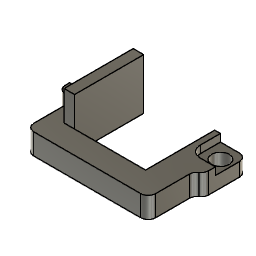
GB DMG - Jack Spacer v15 (Autodesk Fusion 360 design; units mm, degrees)
Autodesk Fusion 360 part; units mm, degrees
sketch "Boceto1" plane through (0, 0, 0) normal (0, 0, 1) x (1, 0, 0)
  line L0 (0, 0) -> (-8.15, 0)
  line L1 (-8.15, 0) -> (-8.15, 6.5)
  line L2 (-8.15, 6.5) -> (-10.45, 6.5)
  line L3 (-10.45, 6.5) -> (-10.45, 12.3)
  line L4 (-10.45, 12.3) -> (-4.75, 12.3)
  line L5 (0, 3.05) -> (-4.75, 3.05)
  line L6 (-4.75, 3.05) -> (-4.75, 12.3)
  line L7 (0, 3.05) -> (0, 0)
  line L8 (4.75, 3.05) -> (4.75, 12.3)
  line L9 (8.15, 6.5) -> (10.45, 6.5)
  line L10 (8.15, 0) -> (8.15, 6.5)
  line L11 (10.45, 12.3) -> (4.75, 12.3)
  line L12 (0, 3.05) -> (4.75, 3.05)
  line L13 (10.45, 6.5) -> (10.45, 12.3)
  line L14 (0, 3.05) -> (0, 0)
  line L15 (0, 0) -> (8.15, 0)
  dimension "d2" = 5.8
  dimension "d3" = 2.3
  dimension "d5" = 8.15
  dimension "d7" = 3.4
  dimension "d8" = 3.05
  dimension "d22" = 9.25
  constraint coincident L0.start L7.end
  constraint horizontal L0
  constraint perpendicular L0 L1
  constraint perpendicular L1 L2
  constraint perpendicular L0 L3
  constraint perpendicular L1 L4
  constraint parallel L4 L5
  constraint perpendicular L4 L6
  constraint perpendicular L0 L7
  constraint symmetric L0.start L7 L14.end
  constraint symmetric L0.end L7 L10.start
  constraint symmetric L1.end L7 L9.start
  constraint symmetric L2.end L7 L9.end
  constraint symmetric L3.end L7 L11.start
  constraint symmetric L5.start L7 L12.start
  constraint symmetric L5.end L7 L8.start
  constraint symmetric L4.end L7 L8.end
  measures "d2" distance of L2.end L3.end
  measures "d3" distance of L1.end L2.end
  measures "d5" distance of L0.start L0.end
  measures "d7" horizontal distance of L1.end L4.end
  measures "d8" distance of L0.start L5.start
  measures "d22" distance of L5.end L4.end
extrude "Extruir1" add sketch "Boceto1" along normal blind 2.8
extrude "Extruir7" cut 1 faces at (10.45, 8.4333, 0.9333) along direction (-1, 0, 0) blind 0.5
sketch "Boceto2" plane through (0, 0, 2.8) normal (0, 0, 1) x (-1, 0, 0)
  line L0 (8.15, 0) -> (-8.15, 0)
  line L1 (-8.15, 0) -> (-8.15, -6.5)
  line L2 (-8.15, -6.5) -> (-9.95, -6.5)
  line L3 (-9.95, -12.3) -> (-4.75, -12.3)
  line L4 (-4.75, -12.3) -> (-4.75, -3.05)
  line L5 (-4.75, -3.05) -> (4.75, -3.05)
  line L6 (4.75, -3.05) -> (4.75, -12.3)
  line L7 (4.75, -12.3) -> (10.45, -12.3)
  line L8 (10.45, -12.3) -> (10.45, -6.5)
  line L9 (10.45, -6.5) -> (8.15, -6.5)
  line L10 (8.15, -6.5) -> (8.15, 0)
  circle A0 centre (8.5, -10.3) radius 1.175
  line L11 (0, -3.05) -> (0, 0)
  line L12 (-9.95, -6.5) -> (-9.95, -12.3)
  line L13 (10.45, -8.1) -> (6.15, -8.1)
  circle A1 centre (-7.5147, -10.3) radius 1.175
  line L14 (-9.95, -8.1) -> (-5.5147, -8.1)
  line L15 (-5.5147, -8.1) -> (-5.5147, -12.3)
  line L16 (6.15, -12.3) -> (6.15, -3.05)
  line L17 (4.75, -3.05) -> (6.15, -3.05)
  point P0 (8.5, -10.3)
  point P1 (-7.5147, -10.3)
  dimension "d13" = 2.35
  dimension "d32" = 2
  dimension "d34" = 1.6
  dimension "d47" = 8.5
  dimension "d49" = 2
  dimension "d50" = 16.0147
  dimension "d51" = 2.35
  dimension "d53" = 2
  dimension "d54" = 1.6
  dimension "d59" = 1.4
  constraint coincident P0 A0.centre
  constraint coincident L8 L13.start
  constraint perpendicular L8 L13
  constraint coincident P1 A1.centre
  constraint coincident L12 L14.start
  constraint perpendicular L12 L14
  constraint coincident L3 L15.end
  constraint perpendicular L3 L15
  constraint coincident L7 L16.start
  constraint perpendicular L7 L16
  constraint coincident L5.end L6.start
  constraint coincident L16 L17.end
  constraint perpendicular L16 L17
  constraint coincident L13.end L16
  measures "d13" diameter of A0
  measures "d32" vertical distance of L6.end P0
  measures "d34" distance of L8.end L13.start
  measures "d47" distance of P0 L11
  measures "d49" vertical distance of L3.start P1
  measures "d50" distance of P0 P1
  measures "d51" diameter of A1
  measures "d53" horizontal distance of P1 L15.end
  measures "d54" distance of L2.end L14.start
  measures "d59" distance of L5.end L16.end
extrude "Extruir8" cut sketch "Boceto2" against normal blind 1 contours L7 L8 L13 L16 | L3 L12 L14 L15 | A0 | A1
extrude "Extruir9" cut sketch "Boceto2" against normal blind 3 contours A0 | A1
extrude "Extruir10" cut 1 faces at (9.95, 8.9667, 0.6) along direction (-1, 0, 0) blind 0.9
extrude "Extruir11" add sketch "Boceto2" along normal blind 4 contours L6 L7 L16 L17
fillet "Empalme1" radius 1.5 1 edges at (5.5147, 8.1, 2.3)
fillet "Empalme2" radius 1 9 edges at (-10.45, 12.3, 0.9) (9.05, 12.3, 0.9) (-10.45, 6.5, 1.4) (9.05, 6.5, 1.4) (-8.15, 0, 1.4) (8.15, 0, 1.4) (-8.15, 6.5, 1.4) (8.15, 6.5, 1.4) (-6.15, 8.1, 2.3)
equation "d14 = d13 + 1 mm"
equation "d23 = d14 + 0.5 mm"
equation "d49 = d32"
equation "d51 = d13"
equation "d52 = 2.00 mm"
equation "d53 = d52"
equation "d54 = d34"
